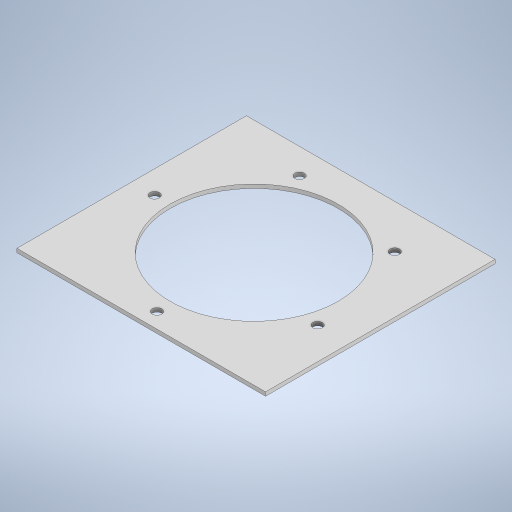
# Autodesk Inventor part: Мотор стенка
Saved by Autodesk Inventor 2023 (Build 270158000, 158)
## iProperties
Created: 2022-05-23
Part Number: Мотор стенка
Material: Типовые
Document SubType Name: Modeling
Designer: User
Density: 1 g/cm^3
Appearance: По умолчанию
Author: User
Autodesk Inventor part; units mm, degrees
ref_plane "YZ Plane" through (0, 0, 0) normal (1, 0, 0) x (0, 1, 0)
ref_plane "XZ Plane" through (0, 0, 0) normal (0, 1, 0) x (-1, 0, 0)
ref_plane "XY Plane" through (0, 0, 0) normal (0, 0, 1) x (1, 0, 0)
sketch "Эскиз1" plane through (0, 0, 0) normal (0, 1, 0) x (-1, 0, 0)
  line L0 (0, 0) -> (130, 0)
  line L1 (130, 0) -> (130, -120)
  line L2 (130, -120) -> (0, -120)
  line L3 (0, -120) -> (0, 0)
  line L4 (0, -60) -> (66, -60)
  circle A0 centre (66, -60) radius 52
  circle A1 centre (118, -60) radius 2.5
  circle A2 centre (16.5955, -43.7767) radius 2.5
  circle A3 centre (64.7729, -8.0145) radius 2.5
  circle A4 centre (88.9135, -106.6795) radius 2.5
  circle A5 centre (29.6669, -97.2009) radius 2.5
  circle A6 centre (66, -60) radius 44
  dimension "d0" = 130
  dimension "d1" = 120
  dimension "d2" = 66
  dimension "d4" = 104
  dimension "d5" = 5
  dimension "d9" = 5
  dimension "d11" = 5
  dimension "d14" = 5
  dimension "d15" = 5
  dimension "d16" = 88
  constraints: 10 end point, 7 centre point, 4 point on circle, 2 coincident, 2 horizontal, 2 parallel, 1 midpoint, 1 perpendicular
  measures "d0" distance of L1.end L2.end
  measures "d1" distance of L0.end L1.end
  measures "d2" distance of L4.start L4.end
  measures "d4" diameter of A0
  measures "d5" diameter of A1
  measures "d9" diameter of A2
  measures "d11" diameter of A3
  measures "d14" diameter of A4
  measures "d15" diameter of A5
  measures "d16" diameter of A6
extrude "Выдавливание1" add sketch "Эскиз1" along normal blind 2 contours L0 L1 L2 L3 | A1 A0 A4 A5 A2 A3
